Autodesk Fusion 360 part; units mm, degrees
(part 2 of 2)
  line L652 (-6.7443, -68.3161) -> (-9.631, -68.3161)
  line L653 (-5.3009, -70.8161) -> (-6.7443, -68.3161)
  line L654 (-1.7956, -76.1733) -> (-0.3522, -73.6733)
  line L655 (-4.6823, -76.1733) -> (-1.7956, -76.1733)
  line L656 (-6.1257, -73.6733) -> (-4.6823, -76.1733)
  line L657 (-4.6823, -71.1733) -> (-6.1257, -73.6733)
  line L658 (-1.7956, -71.1733) -> (-4.6823, -71.1733)
  line L659 (-0.3522, -73.6733) -> (-1.7956, -71.1733)
  line L660 (3.1532, -79.0304) -> (4.5965, -76.5304)
  line L661 (0.2664, -79.0304) -> (3.1532, -79.0304)
  line L662 (-1.177, -76.5304) -> (0.2664, -79.0304)
  line L663 (0.2664, -74.0304) -> (-1.177, -76.5304)
  line L664 (3.1532, -74.0304) -> (0.2664, -74.0304)
  line L665 (4.5965, -76.5304) -> (3.1532, -74.0304)
  line L666 (8.1019, -81.8875) -> (9.5453, -79.3875)
  line L667 (5.2151, -81.8875) -> (8.1019, -81.8875)
  line L668 (3.7718, -79.3875) -> (5.2151, -81.8875)
  line L669 (5.2151, -76.8875) -> (3.7718, -79.3875)
  line L670 (8.1019, -76.8875) -> (5.2151, -76.8875)
  line L671 (9.5453, -79.3875) -> (8.1019, -76.8875)
  line L672 (13.0506, -84.7447) -> (14.494, -82.2447)
  line L673 (10.1638, -84.7447) -> (13.0506, -84.7447)
  line L674 (8.7205, -82.2447) -> (10.1638, -84.7447)
  line L675 (10.1638, -79.7447) -> (8.7205, -82.2447)
  line L676 (13.0506, -79.7447) -> (10.1638, -79.7447)
  line L677 (14.494, -82.2447) -> (13.0506, -79.7447)
  line L678 (17.9993, -87.6018) -> (19.4427, -85.1018)
  line L679 (15.1126, -87.6018) -> (17.9993, -87.6018)
  line L680 (13.6692, -85.1018) -> (15.1126, -87.6018)
  line L681 (15.1126, -82.6018) -> (13.6692, -85.1018)
  line L682 (17.9993, -82.6018) -> (15.1126, -82.6018)
  line L683 (19.4427, -85.1018) -> (17.9993, -82.6018)
  line L684 (22.948, -90.459) -> (24.3914, -87.959)
  line L685 (20.0613, -90.459) -> (22.948, -90.459)
  line L686 (18.6179, -87.959) -> (20.0613, -90.459)
  line L687 (20.0613, -85.459) -> (18.6179, -87.959)
  line L688 (22.948, -85.459) -> (20.0613, -85.459)
  line L689 (24.3914, -87.959) -> (22.948, -85.459)
  line L690 (32.8455, -96.1733) -> (34.2888, -93.6733)
  line L691 (29.9587, -96.1733) -> (32.8455, -96.1733)
  line L692 (28.5153, -93.6733) -> (29.9587, -96.1733)
  line L693 (29.9587, -91.1733) -> (28.5153, -93.6733)
  line L694 (32.8455, -91.1733) -> (29.9587, -91.1733)
  line L695 (34.2888, -93.6733) -> (32.8455, -91.1733)
  line L696 (37.7942, -99.0304) -> (39.2376, -96.5304)
  line L697 (34.9074, -99.0304) -> (37.7942, -99.0304)
  line L698 (33.4641, -96.5304) -> (34.9074, -99.0304)
  line L699 (34.9074, -94.0304) -> (33.4641, -96.5304)
  line L700 (37.7942, -94.0304) -> (34.9074, -94.0304)
  line L701 (39.2376, -96.5304) -> (37.7942, -94.0304)
  line L702 (42.7429, -101.8875) -> (44.1863, -99.3875)
  line L703 (39.8561, -101.8875) -> (42.7429, -101.8875)
  line L704 (38.4128, -99.3875) -> (39.8561, -101.8875)
  line L705 (39.8561, -96.8875) -> (38.4128, -99.3875)
  line L706 (42.7429, -96.8875) -> (39.8561, -96.8875)
  line L707 (44.1863, -99.3875) -> (42.7429, -96.8875)
  line L708 (47.6916, -104.7447) -> (49.135, -102.2447)
  line L709 (44.8049, -104.7447) -> (47.6916, -104.7447)
  line L710 (43.3615, -102.2447) -> (44.8049, -104.7447)
  line L711 (44.8049, -99.7447) -> (43.3615, -102.2447)
  line L712 (47.6916, -99.7447) -> (44.8049, -99.7447)
  line L713 (49.135, -102.2447) -> (47.6916, -99.7447)
  line L714 (52.6403, -107.6018) -> (54.0837, -105.1018)
  line L715 (49.7536, -107.6018) -> (52.6403, -107.6018)
  line L716 (48.3102, -105.1018) -> (49.7536, -107.6018)
  line L717 (49.7536, -102.6018) -> (48.3102, -105.1018)
  line L718 (52.6403, -102.6018) -> (49.7536, -102.6018)
  line L719 (54.0837, -105.1018) -> (52.6403, -102.6018)
  line L720 (57.589, -110.459) -> (59.0324, -107.959)
  line L721 (54.7023, -110.459) -> (57.589, -110.459)
  line L722 (53.2589, -107.959) -> (54.7023, -110.459)
  line L723 (54.7023, -105.459) -> (53.2589, -107.959)
  line L724 (57.589, -105.459) -> (54.7023, -105.459)
  line L725 (59.0324, -107.959) -> (57.589, -105.459)
  line L726 (62.5378, -113.3161) -> (63.9811, -110.8161)
  line L727 (59.651, -113.3161) -> (62.5378, -113.3161)
  line L728 (58.2076, -110.8161) -> (59.651, -113.3161)
  line L729 (59.651, -108.3161) -> (58.2076, -110.8161)
  line L730 (62.5378, -108.3161) -> (59.651, -108.3161)
  line L731 (63.9811, -110.8161) -> (62.5378, -108.3161)
  line L732 (-1.7956, -70.459) -> (-0.3522, -67.959)
  line L733 (-4.6823, -70.459) -> (-1.7956, -70.459)
  line L734 (-6.1257, -67.959) -> (-4.6823, -70.459)
  line L735 (-4.6823, -65.459) -> (-6.1257, -67.959)
  line L736 (-1.7956, -65.459) -> (-4.6823, -65.459)
  line L737 (-0.3522, -67.959) -> (-1.7956, -65.459)
  line L738 (3.1532, -73.3161) -> (4.5965, -70.8161)
  line L739 (0.2664, -73.3161) -> (3.1532, -73.3161)
  line L740 (-1.177, -70.8161) -> (0.2664, -73.3161)
  line L741 (0.2664, -68.3161) -> (-1.177, -70.8161)
  line L742 (3.1532, -68.3161) -> (0.2664, -68.3161)
  line L743 (4.5965, -70.8161) -> (3.1532, -68.3161)
  line L744 (8.1019, -76.1733) -> (9.5453, -73.6733)
  line L745 (5.2151, -76.1733) -> (8.1019, -76.1733)
  line L746 (3.7718, -73.6733) -> (5.2151, -76.1733)
  line L747 (5.2151, -71.1733) -> (3.7718, -73.6733)
  line L748 (8.1019, -71.1733) -> (5.2151, -71.1733)
  line L749 (9.5453, -73.6733) -> (8.1019, -71.1733)
  line L750 (13.0506, -79.0304) -> (14.494, -76.5304)
  line L751 (10.1638, -79.0304) -> (13.0506, -79.0304)
  line L752 (8.7205, -76.5304) -> (10.1638, -79.0304)
  line L753 (10.1638, -74.0304) -> (8.7205, -76.5304)
  line L754 (13.0506, -74.0304) -> (10.1638, -74.0304)
  line L755 (14.494, -76.5304) -> (13.0506, -74.0304)
  line L756 (17.9993, -81.8875) -> (19.4427, -79.3875)
  line L757 (15.1126, -81.8875) -> (17.9993, -81.8875)
  line L758 (13.6692, -79.3875) -> (15.1126, -81.8875)
  line L759 (15.1126, -76.8875) -> (13.6692, -79.3875)
  line L760 (17.9993, -76.8875) -> (15.1126, -76.8875)
  line L761 (19.4427, -79.3875) -> (17.9993, -76.8875)
  line L762 (22.948, -84.7447) -> (24.3914, -82.2447)
  line L763 (20.0613, -84.7447) -> (22.948, -84.7447)
  line L764 (18.6179, -82.2447) -> (20.0613, -84.7447)
  line L765 (20.0613, -79.7447) -> (18.6179, -82.2447)
  line L766 (22.948, -79.7447) -> (20.0613, -79.7447)
  line L767 (24.3914, -82.2447) -> (22.948, -79.7447)
  line L768 (27.8967, -87.6018) -> (29.3401, -85.1018)
  line L769 (25.01, -87.6018) -> (27.8967, -87.6018)
  line L770 (23.5666, -85.1018) -> (25.01, -87.6018)
  line L771 (25.01, -82.6018) -> (23.5666, -85.1018)
  line L772 (27.8967, -82.6018) -> (25.01, -82.6018)
  line L773 (29.3401, -85.1018) -> (27.8967, -82.6018)
  line L774 (32.8455, -90.459) -> (34.2888, -87.959)
  line L775 (29.9587, -90.459) -> (32.8455, -90.459)
  line L776 (28.5153, -87.959) -> (29.9587, -90.459)
  line L777 (29.9587, -85.459) -> (28.5153, -87.959)
  line L778 (32.8455, -85.459) -> (29.9587, -85.459)
  line L779 (34.2888, -87.959) -> (32.8455, -85.459)
  line L780 (37.7942, -93.3161) -> (39.2376, -90.8161)
  line L781 (34.9074, -93.3161) -> (37.7942, -93.3161)
  line L782 (33.4641, -90.8161) -> (34.9074, -93.3161)
  line L783 (34.9074, -88.3161) -> (33.4641, -90.8161)
  line L784 (37.7942, -88.3161) -> (34.9074, -88.3161)
  line L785 (39.2376, -90.8161) -> (37.7942, -88.3161)
  line L786 (42.7429, -96.1733) -> (44.1863, -93.6733)
  line L787 (39.8561, -96.1733) -> (42.7429, -96.1733)
  line L788 (38.4128, -93.6733) -> (39.8561, -96.1733)
  line L789 (39.8561, -91.1733) -> (38.4128, -93.6733)
  line L790 (42.7429, -91.1733) -> (39.8561, -91.1733)
  line L791 (44.1863, -93.6733) -> (42.7429, -91.1733)
  line L792 (47.6916, -99.0304) -> (49.135, -96.5304)
  line L793 (44.8049, -99.0304) -> (47.6916, -99.0304)
  line L794 (43.3615, -96.5304) -> (44.8049, -99.0304)
  line L795 (44.8049, -94.0304) -> (43.3615, -96.5304)
  line L796 (47.6916, -94.0304) -> (44.8049, -94.0304)
  line L797 (49.135, -96.5304) -> (47.6916, -94.0304)
  line L798 (52.6403, -101.8875) -> (54.0837, -99.3875)
  line L799 (49.7536, -101.8875) -> (52.6403, -101.8875)
  line L800 (48.3102, -99.3875) -> (49.7536, -101.8875)
  line L801 (49.7536, -96.8875) -> (48.3102, -99.3875)
  line L802 (52.6403, -96.8875) -> (49.7536, -96.8875)
  line L803 (54.0837, -99.3875) -> (52.6403, -96.8875)
  line L804 (57.589, -104.7447) -> (59.0324, -102.2447)
  line L805 (54.7023, -104.7447) -> (57.589, -104.7447)
  line L806 (53.2589, -102.2447) -> (54.7023, -104.7447)
  line L807 (54.7023, -99.7447) -> (53.2589, -102.2447)
  line L808 (57.589, -99.7447) -> (54.7023, -99.7447)
  line L809 (59.0324, -102.2447) -> (57.589, -99.7447)
  line L810 (62.5378, -107.6018) -> (63.9811, -105.1018)
  line L811 (59.651, -107.6018) -> (62.5378, -107.6018)
  line L812 (58.2076, -105.1018) -> (59.651, -107.6018)
  line L813 (59.651, -102.6018) -> (58.2076, -105.1018)
  line L814 (62.5378, -102.6018) -> (59.651, -102.6018)
  line L815 (63.9811, -105.1018) -> (62.5378, -102.6018)
  line L816 (67.4865, -110.459) -> (68.9299, -107.959)
  line L817 (64.5997, -110.459) -> (67.4865, -110.459)
  line L818 (63.1564, -107.959) -> (64.5997, -110.459)
  line L819 (64.5997, -105.459) -> (63.1564, -107.959)
  line L820 (67.4865, -105.459) -> (64.5997, -105.459)
  line L821 (68.9299, -107.959) -> (67.4865, -105.459)
  line L822 (3.1532, -67.6018) -> (4.5965, -65.1018)
  line L823 (0.2664, -67.6018) -> (3.1532, -67.6018)
  line L824 (-1.177, -65.1018) -> (0.2664, -67.6018)
  line L825 (0.2664, -62.6018) -> (-1.177, -65.1018)
  line L826 (3.1532, -62.6018) -> (0.2664, -62.6018)
  line L827 (4.5965, -65.1018) -> (3.1532, -62.6018)
  line L828 (8.1019, -70.459) -> (9.5453, -67.959)
  line L829 (5.2151, -70.459) -> (8.1019, -70.459)
  line L830 (3.7718, -67.959) -> (5.2151, -70.459)
  line L831 (5.2151, -65.459) -> (3.7718, -67.959)
  line L832 (8.1019, -65.459) -> (5.2151, -65.459)
  line L833 (9.5453, -67.959) -> (8.1019, -65.459)
  line L834 (13.0506, -73.3161) -> (14.494, -70.8161)
  line L835 (10.1638, -73.3161) -> (13.0506, -73.3161)
  line L836 (8.7205, -70.8161) -> (10.1638, -73.3161)
  line L837 (10.1638, -68.3161) -> (8.7205, -70.8161)
  line L838 (13.0506, -68.3161) -> (10.1638, -68.3161)
  line L839 (14.494, -70.8161) -> (13.0506, -68.3161)
  line L840 (17.9993, -76.1733) -> (19.4427, -73.6733)
  line L841 (15.1126, -76.1733) -> (17.9993, -76.1733)
  line L842 (13.6692, -73.6733) -> (15.1126, -76.1733)
  line L843 (15.1126, -71.1733) -> (13.6692, -73.6733)
  line L844 (17.9993, -71.1733) -> (15.1126, -71.1733)
  line L845 (19.4427, -73.6733) -> (17.9993, -71.1733)
  line L846 (22.948, -79.0304) -> (24.3914, -76.5304)
  line L847 (20.0613, -79.0304) -> (22.948, -79.0304)
  line L848 (18.6179, -76.5304) -> (20.0613, -79.0304)
  line L849 (20.0613, -74.0304) -> (18.6179, -76.5304)
  line L850 (22.948, -74.0304) -> (20.0613, -74.0304)
  line L851 (24.3914, -76.5304) -> (22.948, -74.0304)
  line L852 (27.8967, -81.8875) -> (29.3401, -79.3875)
  line L853 (25.01, -81.8875) -> (27.8967, -81.8875)
  line L854 (23.5666, -79.3875) -> (25.01, -81.8875)
  line L855 (25.01, -76.8875) -> (23.5666, -79.3875)
  line L856 (27.8967, -76.8875) -> (25.01, -76.8875)
  line L857 (29.3401, -79.3875) -> (27.8967, -76.8875)
  line L858 (32.8455, -84.7447) -> (34.2888, -82.2447)
  line L859 (29.9587, -84.7447) -> (32.8455, -84.7447)
  line L860 (28.5153, -82.2447) -> (29.9587, -84.7447)
  line L861 (29.9587, -79.7447) -> (28.5153, -82.2447)
  line L862 (32.8455, -79.7447) -> (29.9587, -79.7447)
  line L863 (34.2888, -82.2447) -> (32.8455, -79.7447)
  line L864 (37.7942, -87.6018) -> (39.2376, -85.1018)
  line L865 (34.9074, -87.6018) -> (37.7942, -87.6018)
  line L866 (33.4641, -85.1018) -> (34.9074, -87.6018)
  line L867 (34.9074, -82.6018) -> (33.4641, -85.1018)
  line L868 (37.7942, -82.6018) -> (34.9074, -82.6018)
  line L869 (39.2376, -85.1018) -> (37.7942, -82.6018)
  line L870 (42.7429, -90.459) -> (44.1863, -87.959)
  line L871 (39.8561, -90.459) -> (42.7429, -90.459)
  line L872 (38.4128, -87.959) -> (39.8561, -90.459)
  line L873 (39.8561, -85.459) -> (38.4128, -87.959)
  line L874 (42.7429, -85.459) -> (39.8561, -85.459)
  line L875 (44.1863, -87.959) -> (42.7429, -85.459)
  line L876 (47.6916, -93.3161) -> (49.135, -90.8161)
  line L877 (44.8049, -93.3161) -> (47.6916, -93.3161)
  line L878 (43.3615, -90.8161) -> (44.8049, -93.3161)
  line L879 (44.8049, -88.3161) -> (43.3615, -90.8161)
  line L880 (47.6916, -88.3161) -> (44.8049, -88.3161)
  line L881 (49.135, -90.8161) -> (47.6916, -88.3161)
  line L882 (52.6403, -96.1733) -> (54.0837, -93.6733)
  line L883 (49.7536, -96.1733) -> (52.6403, -96.1733)
  line L884 (48.3102, -93.6733) -> (49.7536, -96.1733)
  line L885 (49.7536, -91.1733) -> (48.3102, -93.6733)
  line L886 (52.6403, -91.1733) -> (49.7536, -91.1733)
  line L887 (54.0837, -93.6733) -> (52.6403, -91.1733)
  line L888 (57.589, -99.0304) -> (59.0324, -96.5304)
  line L889 (54.7023, -99.0304) -> (57.589, -99.0304)
  line L890 (53.2589, -96.5304) -> (54.7023, -99.0304)
  line L891 (54.7023, -94.0304) -> (53.2589, -96.5304)
  line L892 (57.589, -94.0304) -> (54.7023, -94.0304)
  line L893 (59.0324, -96.5304) -> (57.589, -94.0304)
  line L894 (62.5378, -101.8875) -> (63.9811, -99.3875)
  line L895 (59.651, -101.8875) -> (62.5378, -101.8875)
  line L896 (58.2076, -99.3875) -> (59.651, -101.8875)
  line L897 (59.651, -96.8875) -> (58.2076, -99.3875)
  line L898 (62.5378, -96.8875) -> (59.651, -96.8875)
  line L899 (63.9811, -99.3875) -> (62.5378, -96.8875)
  line L900 (67.4865, -104.7447) -> (68.9299, -102.2447)
  line L901 (64.5997, -104.7447) -> (67.4865, -104.7447)
  line L902 (63.1564, -102.2447) -> (64.5997, -104.7447)
  line L903 (64.5997, -99.7447) -> (63.1564, -102.2447)
  line L904 (67.4865, -99.7447) -> (64.5997, -99.7447)
  line L905 (68.9299, -102.2447) -> (67.4865, -99.7447)
  line L906 (72.4352, -107.6018) -> (73.8786, -105.1018)
  line L907 (69.5484, -107.6018) -> (72.4352, -107.6018)
  line L908 (68.1051, -105.1018) -> (69.5484, -107.6018)
  line L909 (69.5484, -102.6018) -> (68.1051, -105.1018)
  line L910 (72.4352, -102.6018) -> (69.5484, -102.6018)
  line L911 (73.8786, -105.1018) -> (72.4352, -102.6018)
  line L912 (8.1019, -64.7447) -> (9.5453, -62.2447)
  line L913 (5.2151, -64.7447) -> (8.1019, -64.7447)
  line L914 (3.7718, -62.2447) -> (5.2151, -64.7447)
  line L915 (5.2151, -59.7447) -> (3.7718, -62.2447)
  line L916 (8.1019, -59.7447) -> (5.2151, -59.7447)
  line L917 (9.5453, -62.2447) -> (8.1019, -59.7447)
  line L918 (13.0506, -67.6018) -> (14.494, -65.1018)
  line L919 (10.1638, -67.6018) -> (13.0506, -67.6018)
  line L920 (8.7205, -65.1018) -> (10.1638, -67.6018)
  line L921 (10.1638, -62.6018) -> (8.7205, -65.1018)
  line L922 (13.0506, -62.6018) -> (10.1638, -62.6018)
  line L923 (14.494, -65.1018) -> (13.0506, -62.6018)
  line L924 (17.9993, -70.459) -> (19.4427, -67.959)
  line L925 (15.1126, -70.459) -> (17.9993, -70.459)
  line L926 (13.6692, -67.959) -> (15.1126, -70.459)
  line L927 (15.1126, -65.459) -> (13.6692, -67.959)
  line L928 (17.9993, -65.459) -> (15.1126, -65.459)
  line L929 (19.4427, -67.959) -> (17.9993, -65.459)
  line L930 (22.948, -73.3161) -> (24.3914, -70.8161)
  line L931 (20.0613, -73.3161) -> (22.948, -73.3161)
  line L932 (18.6179, -70.8161) -> (20.0613, -73.3161)
  line L933 (20.0613, -68.3161) -> (18.6179, -70.8161)
  line L934 (22.948, -68.3161) -> (20.0613, -68.3161)
  line L935 (24.3914, -70.8161) -> (22.948, -68.3161)
  line L936 (27.8967, -76.1733) -> (29.3401, -73.6733)
  line L937 (25.01, -76.1733) -> (27.8967, -76.1733)
  line L938 (23.5666, -73.6733) -> (25.01, -76.1733)
  line L939 (25.01, -71.1733) -> (23.5666, -73.6733)
  line L940 (27.8967, -71.1733) -> (25.01, -71.1733)
  line L941 (29.3401, -73.6733) -> (27.8967, -71.1733)
  line L942 (32.8455, -79.0304) -> (34.2888, -76.5304)
  line L943 (29.9587, -79.0304) -> (32.8455, -79.0304)
  line L944 (28.5153, -76.5304) -> (29.9587, -79.0304)
  line L945 (29.9587, -74.0304) -> (28.5153, -76.5304)
  line L946 (32.8455, -74.0304) -> (29.9587, -74.0304)
  line L947 (34.2888, -76.5304) -> (32.8455, -74.0304)
  line L948 (37.7942, -81.8875) -> (39.2376, -79.3875)
  line L949 (34.9074, -81.8875) -> (37.7942, -81.8875)
  line L950 (33.4641, -79.3875) -> (34.9074, -81.8875)
  line L951 (34.9074, -76.8875) -> (33.4641, -79.3875)
  line L952 (37.7942, -76.8875) -> (34.9074, -76.8875)
  line L953 (39.2376, -79.3875) -> (37.7942, -76.8875)
  line L954 (42.7429, -84.7447) -> (44.1863, -82.2447)
  line L955 (39.8561, -84.7447) -> (42.7429, -84.7447)
  line L956 (38.4128, -82.2447) -> (39.8561, -84.7447)
  line L957 (39.8561, -79.7447) -> (38.4128, -82.2447)
  line L958 (42.7429, -79.7447) -> (39.8561, -79.7447)
  line L959 (44.1863, -82.2447) -> (42.7429, -79.7447)
  line L960 (47.6916, -87.6018) -> (49.135, -85.1018)
  line L961 (44.8049, -87.6018) -> (47.6916, -87.6018)
  line L962 (43.3615, -85.1018) -> (44.8049, -87.6018)
  line L963 (44.8049, -82.6018) -> (43.3615, -85.1018)
  line L964 (47.6916, -82.6018) -> (44.8049, -82.6018)
  line L965 (49.135, -85.1018) -> (47.6916, -82.6018)
  line L966 (52.6403, -90.459) -> (54.0837, -87.959)
  line L967 (49.7536, -90.459) -> (52.6403, -90.459)
  line L968 (48.3102, -87.959) -> (49.7536, -90.459)
  line L969 (49.7536, -85.459) -> (48.3102, -87.959)
  line L970 (52.6403, -85.459) -> (49.7536, -85.459)
  line L971 (54.0837, -87.959) -> (52.6403, -85.459)
  line L972 (57.589, -93.3161) -> (59.0324, -90.8161)
  line L973 (54.7023, -93.3161) -> (57.589, -93.3161)
  line L974 (53.2589, -90.8161) -> (54.7023, -93.3161)
  line L975 (54.7023, -88.3161) -> (53.2589, -90.8161)
  line L976 (57.589, -88.3161) -> (54.7023, -88.3161)
  line L977 (59.0324, -90.8161) -> (57.589, -88.3161)
  line L978 (62.5378, -96.1733) -> (63.9811, -93.6733)
  line L979 (59.651, -96.1733) -> (62.5378, -96.1733)
  line L980 (58.2076, -93.6733) -> (59.651, -96.1733)
  line L981 (59.651, -91.1733) -> (58.2076, -93.6733)
  line L982 (62.5378, -91.1733) -> (59.651, -91.1733)
  line L983 (63.9811, -93.6733) -> (62.5378, -91.1733)
  line L984 (67.4865, -99.0304) -> (68.9299, -96.5304)
  line L985 (64.5997, -99.0304) -> (67.4865, -99.0304)
  line L986 (63.1564, -96.5304) -> (64.5997, -99.0304)
  line L987 (64.5997, -94.0304) -> (63.1564, -96.5304)
  line L988 (67.4865, -94.0304) -> (64.5997, -94.0304)
  line L989 (68.9299, -96.5304) -> (67.4865, -94.0304)
  line L990 (72.4352, -101.8875) -> (73.8786, -99.3875)
  line L991 (69.5484, -101.8875) -> (72.4352, -101.8875)
  line L992 (68.1051, -99.3875) -> (69.5484, -101.8875)
  line L993 (69.5484, -96.8875) -> (68.1051, -99.3875)
  line L994 (72.4352, -96.8875) -> (69.5484, -96.8875)
  line L995 (73.8786, -99.3875) -> (72.4352, -96.8875)
  line L996 (77.3839, -104.7447) -> (78.8273, -102.2447)
  line L997 (74.4972, -104.7447) -> (77.3839, -104.7447)
  line L998 (73.0538, -102.2447) -> (74.4972, -104.7447)
  line L999 (74.4972, -99.7447) -> (73.0538, -102.2447)
  line L1000 (77.3839, -99.7447) -> (74.4972, -99.7447)
  line L1001 (78.8273, -102.2447) -> (77.3839, -99.7447)
  line L1002 (13.0506, -61.8875) -> (14.494, -59.3875)
  line L1003 (10.1638, -61.8875) -> (13.0506, -61.8875)
  line L1004 (8.7205, -59.3875) -> (10.1638, -61.8875)
  line L1005 (10.1638, -56.8875) -> (8.7205, -59.3875)
  line L1006 (13.0506, -56.8875) -> (10.1638, -56.8875)
  line L1007 (14.494, -59.3875) -> (13.0506, -56.8875)
  line L1008 (17.9993, -64.7447) -> (19.4427, -62.2447)
  line L1009 (15.1126, -64.7447) -> (17.9993, -64.7447)
  line L1010 (13.6692, -62.2447) -> (15.1126, -64.7447)
  line L1011 (15.1126, -59.7447) -> (13.6692, -62.2447)
  line L1012 (17.9993, -59.7447) -> (15.1126, -59.7447)
  line L1013 (19.4427, -62.2447) -> (17.9993, -59.7447)
  line L1014 (22.948, -67.6018) -> (24.3914, -65.1018)
  line L1015 (20.0613, -67.6018) -> (22.948, -67.6018)
  line L1016 (18.6179, -65.1018) -> (20.0613, -67.6018)
  line L1017 (20.0613, -62.6018) -> (18.6179, -65.1018)
  line L1018 (22.948, -62.6018) -> (20.0613, -62.6018)
  line L1019 (24.3914, -65.1018) -> (22.948, -62.6018)
  line L1020 (27.8967, -70.459) -> (29.3401, -67.959)
  line L1021 (25.01, -70.459) -> (27.8967, -70.459)
  line L1022 (23.5666, -67.959) -> (25.01, -70.459)
  line L1023 (25.01, -65.459) -> (23.5666, -67.959)
  line L1024 (27.8967, -65.459) -> (25.01, -65.459)
  line L1025 (29.3401, -67.959) -> (27.8967, -65.459)
  line L1026 (32.8455, -73.3161) -> (34.2888, -70.8161)
  line L1027 (29.9587, -73.3161) -> (32.8455, -73.3161)
  line L1028 (28.5153, -70.8161) -> (29.9587, -73.3161)
  line L1029 (29.9587, -68.3161) -> (28.5153, -70.8161)
  line L1030 (32.8455, -68.3161) -> (29.9587, -68.3161)
  line L1031 (34.2888, -70.8161) -> (32.8455, -68.3161)
  line L1032 (37.7942, -76.1733) -> (39.2376, -73.6733)
  line L1033 (34.9074, -76.1733) -> (37.7942, -76.1733)
  line L1034 (33.4641, -73.6733) -> (34.9074, -76.1733)
  line L1035 (34.9074, -71.1733) -> (33.4641, -73.6733)
  line L1036 (37.7942, -71.1733) -> (34.9074, -71.1733)
  line L1037 (39.2376, -73.6733) -> (37.7942, -71.1733)
  line L1038 (42.7429, -79.0304) -> (44.1863, -76.5304)
  line L1039 (39.8561, -79.0304) -> (42.7429, -79.0304)
  line L1040 (38.4128, -76.5304) -> (39.8561, -79.0304)
  line L1041 (39.8561, -74.0304) -> (38.4128, -76.5304)
  line L1042 (42.7429, -74.0304) -> (39.8561, -74.0304)
  line L1043 (44.1863, -76.5304) -> (42.7429, -74.0304)
  line L1044 (47.6916, -81.8875) -> (49.135, -79.3875)
  line L1045 (44.8049, -81.8875) -> (47.6916, -81.8875)
  line L1046 (43.3615, -79.3875) -> (44.8049, -81.8875)
  line L1047 (44.8049, -76.8875) -> (43.3615, -79.3875)
  line L1048 (47.6916, -76.8875) -> (44.8049, -76.8875)
  line L1049 (49.135, -79.3875) -> (47.6916, -76.8875)
  line L1050 (52.6403, -84.7447) -> (54.0837, -82.2447)
  line L1051 (49.7536, -84.7447) -> (52.6403, -84.7447)
  line L1052 (48.3102, -82.2447) -> (49.7536, -84.7447)
  line L1053 (49.7536, -79.7447) -> (48.3102, -82.2447)
  line L1054 (52.6403, -79.7447) -> (49.7536, -79.7447)
  line L1055 (54.0837, -82.2447) -> (52.6403, -79.7447)
  line L1056 (57.589, -87.6018) -> (59.0324, -85.1018)
  line L1057 (54.7023, -87.6018) -> (57.589, -87.6018)
  line L1058 (53.2589, -85.1018) -> (54.7023, -87.6018)
  line L1059 (54.7023, -82.6018) -> (53.2589, -85.1018)
  line L1060 (57.589, -82.6018) -> (54.7023, -82.6018)
  line L1061 (59.0324, -85.1018) -> (57.589, -82.6018)
  line L1062 (62.5378, -90.459) -> (63.9811, -87.959)
  line L1063 (59.651, -90.459) -> (62.5378, -90.459)
  line L1064 (58.2076, -87.959) -> (59.651, -90.459)
  line L1065 (59.651, -85.459) -> (58.2076, -87.959)
  line L1066 (62.5378, -85.459) -> (59.651, -85.459)
  line L1067 (63.9811, -87.959) -> (62.5378, -85.459)
  line L1068 (67.4865, -93.3161) -> (68.9299, -90.8161)
  line L1069 (64.5997, -93.3161) -> (67.4865, -93.3161)
  line L1070 (63.1564, -90.8161) -> (64.5997, -93.3161)
  line L1071 (64.5997, -88.3161) -> (63.1564, -90.8161)
  line L1072 (67.4865, -88.3161) -> (64.5997, -88.3161)
  line L1073 (68.9299, -90.8161) -> (67.4865, -88.3161)
  line L1074 (72.4352, -96.1733) -> (73.8786, -93.6733)
  line L1075 (69.5484, -96.1733) -> (72.4352, -96.1733)
  line L1076 (68.1051, -93.6733) -> (69.5484, -96.1733)
  line L1077 (69.5484, -91.1733) -> (68.1051, -93.6733)
  line L1078 (72.4352, -91.1733) -> (69.5484, -91.1733)
  line L1079 (73.8786, -93.6733) -> (72.4352, -91.1733)
  line L1080 (77.3839, -99.0304) -> (78.8273, -96.5304)
  line L1081 (74.4972, -99.0304) -> (77.3839, -99.0304)
  line L1082 (73.0538, -96.5304) -> (74.4972, -99.0304)
  line L1083 (74.4972, -94.0304) -> (73.0538, -96.5304)
  line L1084 (77.3839, -94.0304) -> (74.4972, -94.0304)
  line L1085 (78.8273, -96.5304) -> (77.3839, -94.0304)
  line L1086 (82.3326, -101.8875) -> (83.776, -99.3875)
  line L1087 (79.4459, -101.8875) -> (82.3326, -101.8875)
  line L1088 (78.0025, -99.3875) -> (79.4459, -101.8875)
  line L1089 (79.4459, -96.8875) -> (78.0025, -99.3875)
  line L1090 (82.3326, -96.8875) -> (79.4459, -96.8875)
  line L1091 (83.776, -99.3875) -> (82.3326, -96.8875)
  line L1092 (17.9993, -59.0304) -> (19.4427, -56.5304)
  line L1093 (15.1126, -59.0304) -> (17.9993, -59.0304)
  line L1094 (13.6692, -56.5304) -> (15.1126, -59.0304)
  line L1095 (15.1126, -54.0304) -> (13.6692, -56.5304)
  line L1096 (17.9993, -54.0304) -> (15.1126, -54.0304)
  line L1097 (19.4427, -56.5304) -> (17.9993, -54.0304)
  line L1098 (22.948, -61.8875) -> (24.3914, -59.3875)
  line L1099 (20.0613, -61.8875) -> (22.948, -61.8875)
  line L1100 (18.6179, -59.3875) -> (20.0613, -61.8875)
  line L1101 (20.0613, -56.8875) -> (18.6179, -59.3875)
  line L1102 (22.948, -56.8875) -> (20.0613, -56.8875)
  line L1103 (24.3914, -59.3875) -> (22.948, -56.8875)
  line L1104 (27.8967, -64.7447) -> (29.3401, -62.2447)
  line L1105 (25.01, -64.7447) -> (27.8967, -64.7447)
  line L1106 (23.5666, -62.2447) -> (25.01, -64.7447)
  line L1107 (25.01, -59.7447) -> (23.5666, -62.2447)
  line L1108 (27.8967, -59.7447) -> (25.01, -59.7447)
  line L1109 (29.3401, -62.2447) -> (27.8967, -59.7447)
  line L1110 (32.8455, -67.6018) -> (34.2888, -65.1018)
  line L1111 (29.9587, -67.6018) -> (32.8455, -67.6018)
  line L1112 (28.5153, -65.1018) -> (29.9587, -67.6018)
  line L1113 (29.9587, -62.6018) -> (28.5153, -65.1018)
  line L1114 (32.8455, -62.6018) -> (29.9587, -62.6018)
  line L1115 (34.2888, -65.1018) -> (32.8455, -62.6018)
  line L1116 (37.7942, -70.459) -> (39.2376, -67.959)
  line L1117 (34.9074, -70.459) -> (37.7942, -70.459)
  line L1118 (33.4641, -67.959) -> (34.9074, -70.459)
  line L1119 (34.9074, -65.459) -> (33.4641, -67.959)
  line L1120 (37.7942, -65.459) -> (34.9074, -65.459)
  line L1121 (39.2376, -67.959) -> (37.7942, -65.459)
  line L1122 (42.7429, -73.3161) -> (44.1863, -70.8161)
  line L1123 (39.8561, -73.3161) -> (42.7429, -73.3161)
  line L1124 (38.4128, -70.8161) -> (39.8561, -73.3161)
  line L1125 (39.8561, -68.3161) -> (38.4128, -70.8161)
  line L1126 (42.7429, -68.3161) -> (39.8561, -68.3161)
  line L1127 (44.1863, -70.8161) -> (42.7429, -68.3161)
  line L1128 (47.6916, -76.1733) -> (49.135, -73.6733)
  line L1129 (44.8049, -76.1733) -> (47.6916, -76.1733)
  line L1130 (43.3615, -73.6733) -> (44.8049, -76.1733)
  line L1131 (44.8049, -71.1733) -> (43.3615, -73.6733)
  line L1132 (47.6916, -71.1733) -> (44.8049, -71.1733)
  line L1133 (49.135, -73.6733) -> (47.6916, -71.1733)
  line L1134 (52.6403, -79.0304) -> (54.0837, -76.5304)
  line L1135 (49.7536, -79.0304) -> (52.6403, -79.0304)
  line L1136 (48.3102, -76.5304) -> (49.7536, -79.0304)
  line L1137 (49.7536, -74.0304) -> (48.3102, -76.5304)
  line L1138 (52.6403, -74.0304) -> (49.7536, -74.0304)
  line L1139 (54.0837, -76.5304) -> (52.6403, -74.0304)
  line L1140 (57.589, -81.8875) -> (59.0324, -79.3875)
  line L1141 (54.7023, -81.8875) -> (57.589, -81.8875)
  line L1142 (53.2589, -79.3875) -> (54.7023, -81.8875)
  line L1143 (54.7023, -76.8875) -> (53.2589, -79.3875)
  line L1144 (57.589, -76.8875) -> (54.7023, -76.8875)
  line L1145 (59.0324, -79.3875) -> (57.589, -76.8875)
  line L1146 (62.5378, -84.7447) -> (63.9811, -82.2447)
  line L1147 (59.651, -84.7447) -> (62.5378, -84.7447)
  line L1148 (58.2076, -82.2447) -> (59.651, -84.7447)
  line L1149 (59.651, -79.7447) -> (58.2076, -82.2447)
  line L1150 (62.5378, -79.7447) -> (59.651, -79.7447)
  line L1151 (63.9811, -82.2447) -> (62.5378, -79.7447)
  line L1152 (67.4865, -87.6018) -> (68.9299, -85.1018)
  line L1153 (64.5997, -87.6018) -> (67.4865, -87.6018)
  line L1154 (63.1564, -85.1018) -> (64.5997, -87.6018)
  line L1155 (64.5997, -82.6018) -> (63.1564, -85.1018)
  line L1156 (67.4865, -82.6018) -> (64.5997, -82.6018)
  line L1157 (68.9299, -85.1018) -> (67.4865, -82.6018)
  line L1158 (72.4352, -90.459) -> (73.8786, -87.959)
  line L1159 (69.5484, -90.459) -> (72.4352, -90.459)
  line L1160 (68.1051, -87.959) -> (69.5484, -90.459)
  line L1161 (69.5484, -85.459) -> (68.1051, -87.959)
  line L1162 (72.4352, -85.459) -> (69.5484, -85.459)
  line L1163 (73.8786, -87.959) -> (72.4352, -85.459)
  line L1164 (77.3839, -93.3161) -> (78.8273, -90.8161)
  line L1165 (74.4972, -93.3161) -> (77.3839, -93.3161)
  line L1166 (73.0538, -90.8161) -> (74.4972, -93.3161)
  line L1167 (74.4972, -88.3161) -> (73.0538, -90.8161)
  line L1168 (77.3839, -88.3161) -> (74.4972, -88.3161)
  line L1169 (78.8273, -90.8161) -> (77.3839, -88.3161)
  line L1170 (82.3326, -96.1733) -> (83.776, -93.6733)
  line L1171 (79.4459, -96.1733) -> (82.3326, -96.1733)
  line L1172 (78.0025, -93.6733) -> (79.4459, -96.1733)
  line L1173 (79.4459, -91.1733) -> (78.0025, -93.6733)
  line L1174 (82.3326, -91.1733) -> (79.4459, -91.1733)
  line L1175 (83.776, -93.6733) -> (82.3326, -91.1733)
  line L1176 (87.2813, -99.0304) -> (88.7247, -96.5304)
  line L1177 (84.3946, -99.0304) -> (87.2813, -99.0304)
  line L1178 (82.9512, -96.5304) -> (84.3946, -99.0304)
  line L1179 (84.3946, -94.0304) -> (82.9512, -96.5304)
  line L1180 (87.2813, -94.0304) -> (84.3946, -94.0304)
  line L1181 (88.7247, -96.5304) -> (87.2813, -94.0304)
  line L1182 (22.948, -56.1733) -> (24.3914, -53.6733)
  line L1183 (20.0613, -56.1733) -> (22.948, -56.1733)
  line L1184 (18.6179, -53.6733) -> (20.0613, -56.1733)
  line L1185 (20.0613, -51.1733) -> (18.6179, -53.6733)
  line L1186 (22.948, -51.1733) -> (20.0613, -51.1733)
  line L1187 (24.3914, -53.6733) -> (22.948, -51.1733)
  line L1188 (27.8967, -59.0304) -> (29.3401, -56.5304)
  line L1189 (25.01, -59.0304) -> (27.8967, -59.0304)
  line L1190 (23.5666, -56.5304) -> (25.01, -59.0304)
  line L1191 (25.01, -54.0304) -> (23.5666, -56.5304)
  line L1192 (27.8967, -54.0304) -> (25.01, -54.0304)
  line L1193 (29.3401, -56.5304) -> (27.8967, -54.0304)
  line L1194 (32.8455, -61.8875) -> (34.2888, -59.3875)
  line L1195 (29.9587, -61.8875) -> (32.8455, -61.8875)
  line L1196 (28.5153, -59.3875) -> (29.9587, -61.8875)
  line L1197 (29.9587, -56.8875) -> (28.5153, -59.3875)
  line L1198 (32.8455, -56.8875) -> (29.9587, -56.8875)
  line L1199 (34.2888, -59.3875) -> (32.8455, -56.8875)
  line L1200 (37.7942, -64.7447) -> (39.2376, -62.2447)
  line L1201 (34.9074, -64.7447) -> (37.7942, -64.7447)
  line L1202 (33.4641, -62.2447) -> (34.9074, -64.7447)
  line L1203 (34.9074, -59.7447) -> (33.4641, -62.2447)
  line L1204 (37.7942, -59.7447) -> (34.9074, -59.7447)
  line L1205 (39.2376, -62.2447) -> (37.7942, -59.7447)
  line L1206 (42.7429, -67.6018) -> (44.1863, -65.1018)
  line L1207 (39.8561, -67.6018) -> (42.7429, -67.6018)
  line L1208 (38.4128, -65.1018) -> (39.8561, -67.6018)
  line L1209 (39.8561, -62.6018) -> (38.4128, -65.1018)
  line L1210 (42.7429, -62.6018) -> (39.8561, -62.6018)
  line L1211 (44.1863, -65.1018) -> (42.7429, -62.6018)
  line L1212 (47.6916, -70.459) -> (49.135, -67.959)
  line L1213 (44.8049, -70.459) -> (47.6916, -70.459)
  line L1214 (43.3615, -67.959) -> (44.8049, -70.459)
  line L1215 (44.8049, -65.459) -> (43.3615, -67.959)
  line L1216 (47.6916, -65.459) -> (44.8049, -65.459)
  line L1217 (49.135, -67.959) -> (47.6916, -65.459)
  line L1218 (52.6403, -73.3161) -> (54.0837, -70.8161)
  line L1219 (49.7536, -73.3161) -> (52.6403, -73.3161)
  line L1220 (48.3102, -70.8161) -> (49.7536, -73.3161)
  line L1221 (49.7536, -68.3161) -> (48.3102, -70.8161)
  line L1222 (52.6403, -68.3161) -> (49.7536, -68.3161)
  line L1223 (54.0837, -70.8161) -> (52.6403, -68.3161)
  line L1224 (57.589, -76.1733) -> (59.0324, -73.6733)
  line L1225 (54.7023, -76.1733) -> (57.589, -76.1733)
  line L1226 (53.2589, -73.6733) -> (54.7023, -76.1733)
  line L1227 (54.7023, -71.1733) -> (53.2589, -73.6733)
  line L1228 (57.589, -71.1733) -> (54.7023, -71.1733)
  line L1229 (59.0324, -73.6733) -> (57.589, -71.1733)
  line L1230 (62.5378, -79.0304) -> (63.9811, -76.5304)
  line L1231 (59.651, -79.0304) -> (62.5378, -79.0304)
  line L1232 (58.2076, -76.5304) -> (59.651, -79.0304)
  line L1233 (59.651, -74.0304) -> (58.2076, -76.5304)
  line L1234 (62.5378, -74.0304) -> (59.651, -74.0304)
  line L1235 (63.9811, -76.5304) -> (62.5378, -74.0304)
  line L1236 (67.4865, -81.8875) -> (68.9299, -79.3875)
  line L1237 (64.5997, -81.8875) -> (67.4865, -81.8875)
  line L1238 (63.1564, -79.3875) -> (64.5997, -81.8875)
  line L1239 (64.5997, -76.8875) -> (63.1564, -79.3875)
  line L1240 (67.4865, -76.8875) -> (64.5997, -76.8875)
  line L1241 (68.9299, -79.3875) -> (67.4865, -76.8875)
  line L1242 (72.4352, -84.7447) -> (73.8786, -82.2447)
  line L1243 (69.5484, -84.7447) -> (72.4352, -84.7447)
  line L1244 (68.1051, -82.2447) -> (69.5484, -84.7447)
  line L1245 (69.5484, -79.7447) -> (68.1051, -82.2447)
  line L1246 (72.4352, -79.7447) -> (69.5484, -79.7447)
  line L1247 (73.8786, -82.2447) -> (72.4352, -79.7447)
  line L1248 (77.3839, -87.6018) -> (78.8273, -85.1018)
  line L1249 (74.4972, -87.6018) -> (77.3839, -87.6018)
  line L1250 (73.0538, -85.1018) -> (74.4972, -87.6018)
  line L1251 (74.4972, -82.6018) -> (73.0538, -85.1018)
  line L1252 (77.3839, -82.6018) -> (74.4972, -82.6018)
  line L1253 (78.8273, -85.1018) -> (77.3839, -82.6018)
  line L1254 (82.3326, -90.459) -> (83.776, -87.959)
  line L1255 (79.4459, -90.459) -> (82.3326, -90.459)
  line L1256 (78.0025, -87.959) -> (79.4459, -90.459)
  line L1257 (79.4459, -85.459) -> (78.0025, -87.959)
  line L1258 (82.3326, -85.459) -> (79.4459, -85.459)
  line L1259 (83.776, -87.959) -> (82.3326, -85.459)
  line L1260 (87.2813, -93.3161) -> (88.7247, -90.8161)
  line L1261 (84.3946, -93.3161) -> (87.2813, -93.3161)
  line L1262 (82.9512, -90.8161) -> (84.3946, -93.3161)
  line L1263 (84.3946, -88.3161) -> (82.9512, -90.8161)
  line L1264 (87.2813, -88.3161) -> (84.3946, -88.3161)
  line L1265 (88.7247, -90.8161) -> (87.2813, -88.3161)
  line L1266 (92.2301, -96.1733) -> (93.6734, -93.6733)
  line L1267 (89.3433, -96.1733) -> (92.2301, -96.1733)
  line L1268 (87.8999, -93.6733) -> (89.3433, -96.1733)
  line L1269 (89.3433, -91.1733) -> (87.8999, -93.6733)
  line L1270 (92.2301, -91.1733) -> (89.3433, -91.1733)
  line L1271 (93.6734, -93.6733) -> (92.2301, -91.1733)
  line L1272 (27.8967, -53.3161) -> (29.3401, -50.8161)
  line L1273 (25.01, -53.3161) -> (27.8967, -53.3161)
  line L1274 (23.5666, -50.8161) -> (25.01, -53.3161)
  line L1275 (25.01, -48.3161) -> (23.5666, -50.8161)
  line L1276 (27.8967, -48.3161) -> (25.01, -48.3161)
  line L1277 (29.3401, -50.8161) -> (27.8967, -48.3161)
  line L1278 (32.8455, -56.1733) -> (34.2888, -53.6733)
  line L1279 (29.9587, -56.1733) -> (32.8455, -56.1733)
  line L1280 (28.5153, -53.6733) -> (29.9587, -56.1733)
  line L1281 (29.9587, -51.1733) -> (28.5153, -53.6733)
  line L1282 (32.8455, -51.1733) -> (29.9587, -51.1733)
  line L1283 (34.2888, -53.6733) -> (32.8455, -51.1733)
  line L1284 (37.7942, -59.0304) -> (39.2376, -56.5304)
  line L1285 (34.9074, -59.0304) -> (37.7942, -59.0304)
  line L1286 (33.4641, -56.5304) -> (34.9074, -59.0304)
  line L1287 (34.9074, -54.0304) -> (33.4641, -56.5304)
  line L1288 (37.7942, -54.0304) -> (34.9074, -54.0304)
  line L1289 (39.2376, -56.5304) -> (37.7942, -54.0304)
  line L1290 (42.7429, -61.8875) -> (44.1863, -59.3875)
  line L1291 (39.8561, -61.8875) -> (42.7429, -61.8875)
  line L1292 (38.4128, -59.3875) -> (39.8561, -61.8875)
  line L1293 (39.8561, -56.8875) -> (38.4128, -59.3875)
  line L1294 (42.7429, -56.8875) -> (39.8561, -56.8875)
  line L1295 (44.1863, -59.3875) -> (42.7429, -56.8875)
  line L1296 (47.6916, -64.7447) -> (49.135, -62.2447)
  line L1297 (44.8049, -64.7447) -> (47.6916, -64.7447)
  line L1298 (43.3615, -62.2447) -> (44.8049, -64.7447)
  line L1299 (44.8049, -59.7447) -> (43.3615, -62.2447)
  line L1300 (47.6916, -59.7447) -> (44.8049, -59.7447)
  line L1301 (49.135, -62.2447) -> (47.6916, -59.7447)
  line L1302 (52.6403, -67.6018) -> (54.0837, -65.1018)
  line L1303 (49.7536, -67.6018) -> (52.6403, -67.6018)
  line L1304 (48.3102, -65.1018) -> (49.7536, -67.6018)
  line L1305 (49.7536, -62.6018) -> (48.3102, -65.1018)
  line L1306 (52.6403, -62.6018) -> (49.7536, -62.6018)
  line L1307 (54.0837, -65.1018) -> (52.6403, -62.6018)
  line L1308 (57.589, -70.459) -> (59.0324, -67.959)
  line L1309 (54.7023, -70.459) -> (57.589, -70.459)
  line L1310 (53.2589, -67.959) -> (54.7023, -70.459)
  line L1311 (54.7023, -65.459) -> (53.2589, -67.959)
  line L1312 (57.589, -65.459) -> (54.7023, -65.459)
  line L1313 (59.0324, -67.959) -> (57.589, -65.459)
  line L1314 (62.5378, -73.3161) -> (63.9811, -70.8161)
  line L1315 (59.651, -73.3161) -> (62.5378, -73.3161)
  line L1316 (58.2076, -70.8161) -> (59.651, -73.3161)
  line L1317 (59.651, -68.3161) -> (58.2076, -70.8161)
  line L1318 (62.5378, -68.3161) -> (59.651, -68.3161)
  line L1319 (63.9811, -70.8161) -> (62.5378, -68.3161)
  line L1320 (67.4865, -76.1733) -> (68.9299, -73.6733)
  line L1321 (64.5997, -76.1733) -> (67.4865, -76.1733)
  line L1322 (63.1564, -73.6733) -> (64.5997, -76.1733)
  line L1323 (64.5997, -71.1733) -> (63.1564, -73.6733)
  line L1324 (67.4865, -71.1733) -> (64.5997, -71.1733)
  line L1325 (68.9299, -73.6733) -> (67.4865, -71.1733)
  line L1326 (72.4352, -79.0304) -> (73.8786, -76.5304)
  line L1327 (69.5484, -79.0304) -> (72.4352, -79.0304)
  line L1328 (68.1051, -76.5304) -> (69.5484, -79.0304)
  line L1329 (69.5484, -74.0304) -> (68.1051, -76.5304)
  line L1330 (72.4352, -74.0304) -> (69.5484, -74.0304)
  line L1331 (73.8786, -76.5304) -> (72.4352, -74.0304)
  line L1332 (77.3839, -81.8875) -> (78.8273, -79.3875)
  line L1333 (74.4972, -81.8875) -> (77.3839, -81.8875)
  line L1334 (73.0538, -79.3875) -> (74.4972, -81.8875)
  line L1335 (74.4972, -76.8875) -> (73.0538, -79.3875)
  line L1336 (77.3839, -76.8875) -> (74.4972, -76.8875)
  line L1337 (78.8273, -79.3875) -> (77.3839, -76.8875)
  line L1338 (82.3326, -84.7447) -> (83.776, -82.2447)
  line L1339 (79.4459, -84.7447) -> (82.3326, -84.7447)
  line L1340 (78.0025, -82.2447) -> (79.4459, -84.7447)
  line L1341 (79.4459, -79.7447) -> (78.0025, -82.2447)
  line L1342 (82.3326, -79.7447) -> (79.4459, -79.7447)
  line L1343 (83.776, -82.2447) -> (82.3326, -79.7447)
  line L1344 (87.2813, -87.6018) -> (88.7247, -85.1018)
  line L1345 (84.3946, -87.6018) -> (87.2813, -87.6018)
  line L1346 (82.9512, -85.1018) -> (84.3946, -87.6018)
  line L1347 (84.3946, -82.6018) -> (82.9512, -85.1018)
  line L1348 (87.2813, -82.6018) -> (84.3946, -82.6018)
  line L1349 (88.7247, -85.1018) -> (87.2813, -82.6018)
  line L1350 (92.2301, -90.459) -> (93.6734, -87.959)
  line L1351 (89.3433, -90.459) -> (92.2301, -90.459)
  line L1352 (87.8999, -87.959) -> (89.3433, -90.459)
  line L1353 (89.3433, -85.459) -> (87.8999, -87.959)
  line L1354 (92.2301, -85.459) -> (89.3433, -85.459)
  line L1355 (93.6734, -87.959) -> (92.2301, -85.459)
  line L1356 (97.1788, -93.3161) -> (98.6222, -90.8161)
  line L1357 (94.292, -93.3161) -> (97.1788, -93.3161)
  line L1358 (92.8487, -90.8161) -> (94.292, -93.3161)
  line L1359 (94.292, -88.3161) -> (92.8487, -90.8161)
  line L1360 (97.1788, -88.3161) -> (94.292, -88.3161)
  line L1361 (98.6222, -90.8161) -> (97.1788, -88.3161)
  point P0 (26.4534, -90.8161)
  dimension "d76" = 2.5
  dimension "d79" = 40
  dimension "d80" = 40
  constraint midpoint L0 L4.start
  constraint midpoint L2 L4.end
  constraint midpoint L3 L5.start
  constraint midpoint L4 P0
  constraint coincident P0 L5.end
  constraint midpoint L7 L12.start
  constraint midpoint L9 L13.start
  constraint midpoint L6 L14.end
  constraint midpoint L10 L15.end
  constraint midpoint L11 L16.end
  constraint midpoint L8 L17.end
  measures "d76" distance of P0 L11
extrude "Extrude3'" add sketch "Sketch16" along normal blind 1 contours L0 L3 L4 L5 L6 L11 L354 L358 L359 L363 L364 L365 L438 L439 L442 L443 L450 L452 L453 L454 L455 L459 L460 L461 L522 L523 L526 L527 L546 L548 L549 L550 L551 L555 L556 L606 L607 L610 L611 L637 L638 L639 L640 L715 L716 L717 L718 L780 L781 L782 L799 L800 L801 L802 L876 L877 L878 L883 L884 L885 L886 | L0 L1 L2 L4 L7 L8 L9 L492 L493 L496 L497 L501 L502 L503 L576 L577 L580 L581 L597 L598 L599 L660 L661 L664 L665 L738 L739 L742 L743 L783 L784 L785 L822 L823 L828 L829 L830 L831 L833 L879 L880 L881 L918 L919 L920 L924 L925 L926 L927 L929 L967 L968 L969 L970 L1014 L1015 L1016 L1020 L1021 L1022 L1023 L1025 L1051 L1052 L1053 L1054 L1110 L1111 L1112 L1116 L1117 L1118 L1119 L1121 L1135 L1136 L1137 L1138 L1206 L1207 L1208 L1212 L1213 L1214 L1215 L1217 L1219 L1220 L1221 L1222 L1303 L1304 | L2 L3 L4 L5 L10 L11 L76 L77 L156 L157 L160 L161 L162 L164 L165 L166 L167 L171 L172 L173 L240 L241 L244 L245 L258 L260 L261 L262 L263 L267 L268 L269 L324 L325 L328 L329 L356 L357 L358 L408 L409 L412 L413 L439 L440 L441 L442 L498 L499 L500 L523 L524 L525 L526 L594 L595 L596 L607 L608 L609 L610 sketch seen with x (1, 0, 0) y (0, 1, 0) z (0, 0, 1) at (-3.2702, -79.3076, 21.7435) bodies 4 in component "Component''"
extrude "Extrude4'" cut 1 faces at (31.9665, 3.0586, 30.2652) along direction (0, 0, -1) blind 2 on bodies 4 bodies 4 in component "Component''"
extrude "Extrude5'" add 1 faces at (31.4665, 36.3586, 24.2652) along direction (0, 0, -1) blind 2 on bodies 4 bodies 4 in component "Component''"
extrude "Extrude6'" add 1 faces at (23.9543, 36.3586, 28.2652) along direction (0, 0, 1) blind 1 on bodies 4 bodies 4 in component "Component''"
sketch "Sketch17" plane through (0, 0, 2.2652) normal (0, 0, 1) x (-1, 0, 0)
sketch "Sketch18" plane through (0, 0, 2.2652) normal (0, 0, 1) x (-1, 0, 0)
sketch "Sketch19" plane through (0, 0, 2.2652) normal (0, 0, 1) x (-1, 0, 0)
component "Component" placed x (1, 0, 0) y (0, -1, 0) z (0, 0, -1) at (-0.0668, 33.7586, 2.2652)
component "Component''" placed x (1, 0, 0) y (0, 1, 0) z (0, 0, 1) at (3.2702, 79.3076, -21.7435)
